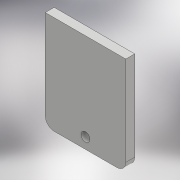
# Autodesk Inventor part: bolsillop2
Saved by Autodesk Inventor 2017 (Build 210142000, 142)
## iProperties
Created: 2018-06-14
Part Number: bolsillop2
Material: Generic
Document SubType Name: Modeling
Designer: Carolina Lema
Density: 1 g/cm^3
Appearance: Default
Author: Carolina Lema
Autodesk Inventor part; units mm, degrees
ref_plane "YZ Plane" through (0, 0, 0) normal (1, 0, 0) x (0, 1, 0)
ref_plane "XZ Plane" through (0, 0, 0) normal (0, 1, 0) x (-1, 0, 0)
ref_plane "XY Plane" through (0, 0, 0) normal (0, 0, 1) x (1, 0, 0)
sketch "Sketch1" plane through (0, 0, 0) normal (0, 1, 0) x (-1, 0, 0)
  line L0 (0, 0) -> (-18, 0)
  line L1 (-18, 0) -> (-18, -22)
  line L2 (-18, -22) -> (0, -22)
  line L3 (0, -22) -> (0, 0)
  line L4 (-1.5, -20.5) -> (2.5, -20.5) construction
  circle A0 centre (-9, -19.8358) radius 1.5
  line L5 (-1, -20.5) -> (-7.6551, -20.5)
  line L6 (-1, -20.5) -> (-1, -1.5)
  line L7 (-1, -1.5) -> (-1, -1)
  line L8 (-1, -1) -> (-17, -1)
  line L9 (-17, -1) -> (-17, -20.5)
  line L10 (-1, -1) -> (-17, -1)
  line L11 (-17, -1) -> (-17, -20.5)
  line L12 (-1, -20.5) -> (-1, -1)
  line L13 (-10.3449, -20.5) -> (-17, -20.5)
  point P0 (0, 0)
  point P1 (-15.5, -20.5)
  dimension "d0" = 18
  dimension "d1" = 22
  dimension "d2" = 3
  dimension "d3" = 0.5
  dimension "d4" = 16
  constraints: 28 end point, 4 horizontal, 4 parallel, 4 point on line, 3 perpendicular, 2 point on circle, 1 centre point, 1 vertical
  measures "d0" distance of L3.start L1.end
  measures "d1" distance of L1.end L1.start
  measures "d2" diameter of A0
  measures "d3" distance of L6.end L12.end
  measures "d4" distance of L12.end L9.start
extrude "Extrusion1" add sketch "Sketch1" along normal blind 2 contours L3 L2 L1 L0 | A0 L13 L9 L8 L7 L6 L5
sketch "Sketch8" plane through (0, 2, 0) normal (0, 1, 0) x (1, 0, 0)
  circle A0 centre (9, 19.8358) radius 1.5 projected
  circle A1 centre (9, 19.8358) radius 1.5 projected
  line L0 (0, 0) -> (18, 0) projected
  line L1 (18, 0) -> (18, 22) projected
  line L2 (18, 22) -> (0, 22) projected
  line L3 (0, 22) -> (0, 0) projected
extrude "Extrusion5" add sketch "Sketch8" against normal blind 2 contours A0
sketch "Sketch9" plane through (0, 2, 0) normal (0, 1, 0) x (1, 0, 0)
  line L0 (0, 0) -> (18, 0) projected
  line L1 (18, 0) -> (18, 22) projected
  line L2 (18, 22) -> (0, 22) projected
  line L3 (0, 22) -> (0, 0) projected
  line L4 (18, 22) -> (18, 17.1361)
  line L5 (15, 16) -> (3, 16)
  line L6 (0, 17.1361) -> (0, 22)
  arc A0 (0, 19) -> (3, 16) centre (3, 19) ccw
  arc A1 (15, 16) -> (18, 19) centre (15, 19) ccw
  line L7 (15, 16) -> (3, 16)
  arc A2 (0, 19) -> (3, 16) centre (3, 19) ccw
  arc A3 (15, 16) -> (18, 19) centre (15, 19) ccw
  line L8 (15, 14.1361) -> (3, 14.1361)
  arc A4 (0, 17.1361) -> (3, 14.1361) centre (3, 17.1361) ccw
  arc A5 (15, 14.1361) -> (18, 17.1361) centre (15, 17.1361) ccw
  line L9 (15, 14.1361) -> (3, 14.1361)
  arc A6 (0, 17.1361) -> (3, 14.1361) centre (3, 17.1361) ccw
  arc A7 (15, 14.1361) -> (18, 17.1361) centre (15, 17.1361) ccw
  circle A8 centre (9, 19.568) radius 2
  dimension "d19" = 4
  constraints: 16 point on circle, 12 end point, 10 tangent, 9 centre point, 2 point on line, 1 parallel
  measures "d19" diameter of A8
extrude "Extrusion6" cut sketch "Sketch9" against normal blind 0.5 contours L3 A4 L8 A5 L1 L0 | L3 L2 L1 A1 L5 A0
sketch "Sketch11" plane through (0, 0, 0) normal (0, -1, 0) x (1, 0, 0)
  line L0 (1.5, -20.5) -> (16.5, -20.5)
  line L1 (16.5, -20.5) -> (16.5, -1.5)
  line L2 (18, -17.1361) -> (18, 0)
  line L3 (0, -22) -> (18, -22)
  line L4 (0, -22) -> (18, -22)
  line L5 (18, -22) -> (18, 0)
  line L6 (16.5, -1.5) -> (1.5, -1.5)
  line L7 (0, -19) -> (0, -22)
  line L8 (1.5, -1.5) -> (1.5, -20.5)
  line L9 (0, 0) -> (0, -22)
  line L10 (0, 0) -> (0, -17.1361)
  line L11 (0, 0) -> (0, -17.1361)
  line L12 (18, -22) -> (18, -19)
  line L13 (18, 0) -> (0, 0) projected
  line L14 (18, 0) -> (0, 0)
  line L15 (0, 0) -> (18, 0)
  line L16 (18, 0) -> (18, -22)
  line L17 (18, -22) -> (0, -22)
  line L18 (0, -22) -> (0, 0)
  line L19 (16.5, -1.5) -> (1.5, -1.5)
  line L20 (1.5, -1.5) -> (1.5, -20.5)
  line L21 (1.5, -20.5) -> (16.5, -20.5)
  line L22 (16.5, -20.5) -> (16.5, -1.5)
  constraints: 44 end point, 4 parallel, 3 horizontal, 2 perpendicular
extrude "Extrusion7" add sketch "Sketch11" against normal blind 2
sketch "Sketch12" plane through (0, 2, 0) normal (0, 1, 0) x (1, 0, 0)
  arc A0 (7.2304, 20.5) -> (10.7696, 20.5) centre (9, 19.568) ccw projected
  circle A1 centre (9, 19.568) radius 1
  point P0 (0, 0)
  dimension "d28" = 2
  constraints: 1 centre point, 1 coincident
  measures "d28" diameter of A1
extrude "Extrusion8" cut sketch "Sketch12" against normal blind 2
fillet "Fillet1" radius 2 2 edges at (0, 1, -22) (18, 1, -22)
body "Solid1"
